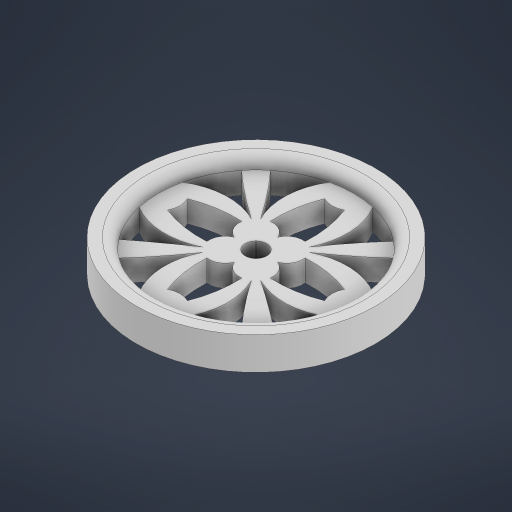
# Autodesk Inventor part: Hjul_Rev1
Saved by Autodesk Inventor 2024 (Build 280153000, 153)
## iProperties
Created: 2023-10-04
Part Number: Hjul_Rev1
Material: Generic
Document SubType Name: Modeling
Designer: 21guslof
Density: 1 g/cm^3
Appearance: Default
Author: 21guslof
Autodesk Inventor part; units mm, degrees
ref_plane "YZ Plane" through (0, 0, 0) normal (1, 0, 0) x (0, 1, 0)
ref_plane "XZ Plane" through (0, 0, 0) normal (0, 1, 0) x (-1, 0, 0)
ref_plane "XY Plane" through (0, 0, 0) normal (0, 0, 1) x (1, 0, 0)
sketch "Sketch1" plane through (0, 0, 0) normal (0, 1, 0) x (-1, 0, 0)
  circle A0 centre (0, 0) radius 2.5
  circle A1 centre (0, 0) radius 5
  circle A2 centre (0, 0) radius 22.5
  circle A3 centre (0, 0) radius 27.5
  arc A4 (0, 5) -> (0, -22.5) centre (21.25, -8.75) ccw
  arc A5 (0, -22.5) -> (0, 5) centre (-21.25, -8.75) ccw
  arc A6 (-5, 0) -> (22.5, 0) centre (8.75, 21.25) ccw
  arc A7 (22.5, 0) -> (-5, 0) centre (8.75, -21.25) ccw
  arc A8 (0, -5) -> (0, 22.5) centre (-21.25, 8.75) ccw
  arc A9 (0, 22.5) -> (0, -5) centre (21.25, 8.75) ccw
  arc A10 (5, 0) -> (-22.5, 0) centre (-8.75, -21.25) ccw
  arc A11 (-22.5, 0) -> (5, 0) centre (-8.75, 21.25) ccw
  circle A12 centre (-22.5, 0) radius 5
  circle A13 centre (0, -22.5) radius 5
  circle A14 centre (22.5, 0) radius 5
  circle A15 centre (0, 22.5) radius 5
  arc A16 (-4.969, 21.9444) -> (-1.7705, 1.7705) centre (8.4478, 13.7311) ccw
  arc A17 (1.7705, 1.7705) -> (4.969, 21.9444) centre (-8.4478, 13.7311) ccw
  arc A18 (4.969, -21.9444) -> (1.7705, -1.7705) centre (-8.4478, -13.7311) ccw
  arc A19 (-1.7705, -1.7705) -> (-4.969, -21.9444) centre (8.4478, -13.7311) ccw
  arc A20 (21.9444, 4.969) -> (1.7705, 1.7705) centre (13.7311, -8.4478) ccw
  arc A21 (1.7705, -1.7705) -> (21.9444, -4.969) centre (13.7311, 8.4478) ccw
  arc A22 (-1.7705, 1.7705) -> (-21.9444, 4.969) centre (-13.7311, -8.4478) ccw
  arc A23 (-21.9444, -4.969) -> (-1.7705, -1.7705) centre (-13.7311, 8.4478) ccw
  circle A24 centre (-3.5128, 3.5128) radius 3.8147
  circle A25 centre (-3.5128, -3.5128) radius 3.8147
  circle A26 centre (3.5128, -3.5128) radius 3.8147
  circle A27 centre (3.5128, 3.5128) radius 3.8147
  arc A28 (-3.5128, -3.5128) -> (-17.5, -14.1421) centre (54.0041, -93.7172) ccw
  arc A29 (-14.1421, -17.5) -> (-3.5128, -3.5128) centre (-93.7172, 54.0041) ccw
  arc A30 (17.5, -14.1421) -> (3.5128, -3.5128) centre (-54.0041, -93.7172) ccw
  arc A31 (3.5128, -3.5128) -> (14.1421, -17.5) centre (93.7172, 54.0041) ccw
  arc A32 (3.5128, 3.5128) -> (17.8243, 13.7311) centre (-104.907, 170.494) ccw
  arc A33 (14.1421, 17.5) -> (3.5128, 3.5128) centre (93.7172, -54.0041) ccw
  arc A34 (-3.5128, 3.5128) -> (-14.1421, 17.5) centre (-93.7172, -54.0041) ccw
  arc A35 (-17.8243, 13.7311) -> (-3.5128, 3.5128) centre (104.907, 170.494) ccw
  point P0 (3.5128, -3.5128)
  point P1 (3.5503, -3.5207)
  point P2 (3.5207, -3.5503)
  point P3 (7.2938, 4.0186)
  point P4 (18.0544, 2.2883)
  point P5 (18.0544, -2.2883)
  point P6 (7.2938, -4.0186)
  point P7 (-3.5128, -3.5128)
  point P8 (-3.5207, -3.5503)
  point P9 (-3.5503, -3.5207)
  point P10 (-18.0544, 2.2883)
  point P11 (-7.2938, 4.0186)
  point P12 (-7.2938, -4.0186)
  point P13 (-18.0544, -2.2883)
  point P14 (-1.7751, -1.7604)
  point P15 (-1.7751, 1.7604)
  point P16 (-1.7604, 1.7751)
  point P17 (1.7604, 1.7751)
  point P18 (1.7751, 1.7604)
  point P19 (1.7751, -1.7604)
  point P20 (1.7604, -1.7751)
  point P21 (-1.7604, -1.7751)
  point P22 (2.2883, 18.0544)
  point P23 (4.0186, 7.2938)
  point P24 (0, 5)
  point P25 (-4.0186, 7.2938)
  point P26 (-2.2883, 18.0544)
  point P27 (4.0186, -7.2938)
  point P28 (2.2883, -18.0544)
  point P29 (-2.2883, -18.0544)
  point P30 (-4.0186, -7.2938)
  point P31 (-6.6922, -5.6207)
  point P32 (-5.6207, -6.6922)
  point P33 (5.6207, -6.6922)
  point P34 (6.6922, -5.6207)
  point P35 (6.6922, 5.6207)
  point P36 (5.6207, 6.6922)
  point P37 (-5.6207, 6.6922)
  point P38 (-6.6922, 5.6207)
  dimension "d2" = 45
  dimension "d0" = 5
  dimension "d1" = 10
  dimension "d3" = 55
  constraints: 76 point on circle, 31 centre point, 8 coincident, 34 other
  measures "d0" diameter of A0
  measures "d1" diameter of A1
  measures "d3" diameter of A3
extrude "Extrusion1" add sketch "Sketch1" along normal blind 5 contours A5 A27 A0 | A8 A26 A27 A5 | A0 A26 A8 | A0 A5 A10 A8 A26 | A27 A5 A11 A8 A0 | A27 A11 A5 | A8 A10 A26 | A11 A1 A6 A5 | A5 A18 A11 | A10 A8 A7 A1 | A26 A6 A1 | A1 A7 A27 | A10 A17 A8 | A0 A24 A7 A5 A10 | A20 A17 | A5 A7 A20 | A11 A8 A6 A25 A0 | A21 A6 A8 | A18 A21 | A31 A1 A5 | A5 A1 A8 A6 | A21 A1 A18 | A30 A1 A21 | A6 A1 A30 | A18 A1 A31 | A7 A32 A1 | A1 A32 A27 A7 | A6 A26 A30 A1 | A7 A5 A1 A8 | A33 A1 A17 | A17 A1 A20 | A20 A1 A32 | A8 A1 A33 | A0 A7 A24 | A7 A24 A5 | A25 A6 A0 | A8 A25 A6 | A5 A26 A1 | A1 A31 A26 A5 | A18 A31 A1 | A1 A21 A26 A18 | A1 A30 A21 | A1 A20 A32 | A27 A20 A14 A7 | A6 A14 A21 A26 | A8 A27 A33 A1 | A1 A27 A8 | A17 A27 A20 A1 | A1 A33 A17 | A10 A27 A24 A7 | A0 A27 A10 | A4 A10 A9 A1 | A27 A10 A4 | A1 A9 A24 | A11 A26 A0 | A6 A25 A26 A11 | A25 A4 A1 | A1 A4 A11 A9 | A9 A11 A26 | A26 A18 A13 A5 | A26 A30 A2 A31 | A27 A33 A2 A32 | A14 A2 A7 | A7 A6 A14 | A6 A2 A14 | A0 A26 A11 A9 A6 | A7 A4 A10 A27 A0 | A8 A15 A17 A27 | A9 A34 A1 | A1 A34 A24 A9 | A4 A22 A10 | A24 A16 A15 A9 | A4 A25 A29 A1 | A1 A29 A4 | A11 A23 A9 | A4 A13 A19 A25 | A13 A2 A5 | A5 A4 A13 | A9 A25 A0 | A0 A24 A4 | A4 A24 A25 A9 | A9 A6 A4 A24 A0 | A0 A25 A9 A7 A4 | A19 A4 A6 | A23 A19 | A7 A9 A16 | A16 A22 | A15 A9 A8 | A8 A2 A15 | A34 A16 A1 | A1 A16 A34 | A9 A7 A1 A10 | A22 A1 A16 | A35 A1 A22 | A10 A1 A35 | A15 A2 A9 | A16 A1 A22 A24 | A24 A35 A2 A34 | A29 A19 A1 | A1 A19 A29 | A11 A1 A6 A4 | A28 A1 A11 | A19 A1 A23 | A23 A1 A28 | A4 A2 A13 | A25 A23 A1 A19 | A29 A2 A28 A25 | A4 A6 A24 | A25 A7 A9 | A10 A24 A35 A1 | A1 A24 A10 | A1 A35 A22 | A24 A10 A12 A22 | A11 A25 A1 | A1 A28 A25 A11 | A23 A28 A1 | A23 A12 A11 A25 | A12 A10 A2 | A2 A11 A12 | A12 A11 A10 picked at (3.6592, 0.0793) picked at (-0.0899, 3.8712) picked at (-0.0899, -3.8712) picked at (-3.6592, -0.0793)
sketch "Sketch2" plane through (0, 0, 0) normal (0, -1, 0) x (1, 0, 0)
  circle A0 centre (0, 0) radius 22.5
  circle A1 centre (0, 0) radius 27.5
  dimension "d6" = 55
  constraints: 2 centre point, 2 coincident
  measures "d6" diameter of A1
extrude "Extrusion2" add sketch "Sketch2" against normal blind 7.5
fillet "Fillet1" radius 2.5 1 edges at (-22.5, 7.5, 0)
body "Solid1"
